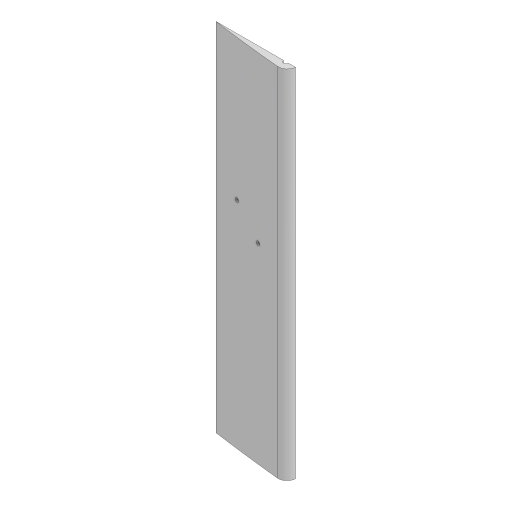
# Autodesk Inventor part: 5P.00.03.01-IB-VTP-Rudder-Right
Saved by Autodesk Inventor 2024.3 (Build 283343000, 343)
## iProperties
Created: 2024-11-01
Part Number: 5P.00.03.01-IB-VTP-Rudder-Right
Material: Generic
Document SubType Name: Modeling
Designer: inigo
Density: 1 g/cm^3
Appearance: Default
Author: inigo
Autodesk Inventor part; units mm, degrees
sketch "Sketch9" plane through (0, 0, 0) normal (0, 1, 0) x (-1, 0, 0)
  spline S0 degree 4 poles (158.6, 0) (158.582, 0.0027) (158.4943, 0.0152) (158.3472, 0.0367) (158.0986, 0.0728) (157.8372, 0.1103) (157.5162, 0.1567) (157.1379, 0.2109) (156.7024, 0.273) (156.2099, 0.3431) (155.661, 0.4204) (155.0564, 0.5055) (154.3967, 0.5974) (153.6823, 0.6963) (152.9144, 0.8018) (152.0931, 0.9136) (151.2197, 1.0314) (150.2949, 1.1553) (149.3195, 1.2842) (148.2947, 1.4185) (147.2214, 1.5576) (146.1008, 1.7014) (144.9336, 1.8489) (143.7214, 2.0008) (142.465, 2.156) (141.166, 2.3142) (139.8256, 2.4755) (138.445, 2.6392) (137.0256, 2.8051) (135.5689, 2.9729) (134.0761, 3.1422) (132.5489, 3.3123) (130.9887, 3.4837) (129.3972, 3.6552) (127.7758, 3.827) (126.126, 3.9983) (124.4499, 4.1692) (122.7486, 4.3392) (121.024, 4.5076) (119.2779, 4.6746) (117.5118, 4.8392) (115.7279, 5.0016) (113.9273, 5.1612) (112.1123, 5.3173) (110.2844, 5.47) (108.4455, 5.6184) (106.5976, 5.7628) (104.7421, 5.9018) (102.8813, 6.0361) (101.0167, 6.1642) (99.1503, 6.2867) (97.2839, 6.4023) (95.4193, 6.511) (93.5585, 6.6124) (91.703, 6.7063) (89.8551, 6.7915) (88.0161, 6.8687) (86.1882, 6.9365) (84.3732, 6.9953) (82.5726, 7.0442) (80.7886, 7.0832) (79.0224, 7.1119) (77.2764, 7.1298) (75.5517, 7.1371) (73.8503, 7.133) (72.1741, 7.1177) (70.5243, 7.091) (68.9027, 7.0524) (67.3112, 7.0021) (65.7508, 6.94) (64.2236, 6.8657) (62.7307, 6.7798) (61.2739, 6.6817) (59.8543, 6.5718) (58.4735, 6.4501) (57.133, 6.3171) (55.8338, 6.1722) (54.5772, 6.0162) (53.3648, 5.8493) (52.1973, 5.6715) (51.0764, 5.483) (50.0027, 5.2845) (48.9775, 5.0759) (48.0018, 4.858) (47.0765, 4.6308) (46.2025, 4.3948) (45.3805, 4.1502) (44.6117, 3.8978) (43.8963, 3.6374) (43.2353, 3.3698) (42.6292, 3.095) (42.0785, 2.8136) (41.5834, 2.526) (41.1451, 2.2317) (40.7628, 1.9317) (40.4377, 1.6254) (40.1698, 1.3127) (39.9596, 0.9936) (39.8087, 0.6678) (39.7177, 0.3364) (39.6875, 0) (39.7177, -0.3364) (39.8087, -0.6678) (39.9596, -0.9936) (40.1698, -1.3127) (40.4377, -1.6254) (40.7628, -1.9317) (41.1451, -2.2317) (41.5834, -2.526) (42.0785, -2.8136) (42.6292, -3.095) (43.2353, -3.3698) (43.8963, -3.6374) (44.6117, -3.8978) (45.3805, -4.1502) (46.2025, -4.3948) (47.0765, -4.6308) (48.0018, -4.858) (48.9775, -5.0759) (50.0027, -5.2845) (51.0764, -5.483) (52.1973, -5.6715) (53.3648, -5.8493) (54.5772, -6.0162) (55.8338, -6.1722) (57.133, -6.3171) (58.4735, -6.4501) (59.8543, -6.5718) (61.2739, -6.6817) (62.7307, -6.7798) (64.2236, -6.8657) (65.7508, -6.94) (67.3112, -7.0021) (68.9027, -7.0524) (70.5243, -7.091) (72.1741, -7.1177) (73.8503, -7.133) (75.5517, -7.1371) (77.2764, -7.1298) (79.0224, -7.1119) (80.7886, -7.0832) (82.5726, -7.0442) (84.3732, -6.9953) (86.1882, -6.9365) (88.0161, -6.8687) (89.8551, -6.7915) (91.703, -6.7063) (93.5585, -6.6124) (95.4193, -6.511) (97.2839, -6.4023) (99.1503, -6.2867) (101.0167, -6.1642) (102.8813, -6.0361) (104.7421, -5.9018) (106.5976, -5.7628) (108.4455, -5.6184) (110.2844, -5.47) (112.1123, -5.3173) (113.9273, -5.1612) (115.7279, -5.0016) (117.5118, -4.8392) (119.2779, -4.6746) (121.024, -4.5076) (122.7486, -4.3392) (124.4499, -4.1692) (126.126, -3.9983) (127.7758, -3.827) (129.3972, -3.6552) (130.9887, -3.4837) (132.5489, -3.3123) (134.0761, -3.1422) (135.5689, -2.9729) (137.0256, -2.8051) (138.445, -2.6392) (139.8256, -2.4755) (141.166, -2.3142) (142.465, -2.156) (143.7214, -2.0008) (144.9336, -1.8489) (146.1008, -1.7014) (147.2214, -1.5576) (148.2947, -1.4185) (149.3195, -1.2842) (150.2949, -1.1553) (151.2197, -1.0314) (152.0931, -0.9136) (152.9144, -0.8018) (153.6823, -0.6963) (154.3967, -0.5974) (155.0564, -0.5055) (155.661, -0.4204) (156.2099, -0.3431) (156.7024, -0.273) (157.1379, -0.2109) (157.5162, -0.1567) (157.8372, -0.1103) (158.0986, -0.0728) (158.3472, -0.0367) (158.4943, -0.0152) (158.582, -0.0027) (158.6, 0) knots 0 0 0 0 0 0.003305 0.005251 0.007517 0.010057 0.012844 0.015853 0.019069 0.022477 0.026064 0.029821 0.033738 0.037807 0.04202 0.046371 0.050853 0.05546 0.060186 0.065027 0.069976 0.07503 0.080184 0.085434 0.090774 0.096201 0.101711 0.1073 0.112964 0.118699 0.124501 0.130368 0.136295 0.142278 0.148315 0.154402 0.160535 0.166711 0.172927 0.179179 0.185465 0.19178 0.198121 0.204486 0.210871 0.217273 0.223689 0.230115 0.236548 0.242985 0.249423 0.255859 0.262289 0.268711 0.275121 0.281516 0.287892 0.294248 0.300579 0.306882 0.313155 0.319394 0.325595 0.331757 0.337875 0.343946 0.349967 0.355935 0.361846 0.367698 0.373486 0.379209 0.384861 0.390441 0.395943 0.401366 0.406705 0.411957 0.417118 0.422185 0.427153 0.432019 0.436778 0.441428 0.445964 0.450381 0.454676 0.458845 0.462884 0.466789 0.470556 0.474184 0.477671 0.481017 0.484224 0.487301 0.490258 0.493116 0.495899 0.498638 0.501362 0.504101 0.506884 0.509742 0.512699 0.515776 0.518983 0.522329 0.525816 0.529444 0.533211 0.537116 0.541155 0.545324 0.549619 0.554036 0.558572 0.563222 0.567981 0.572847 0.577815 0.582882 0.588043 0.593295 0.598634 0.604057 0.609559 0.615139 0.620791 0.626514 0.632302 0.638154 0.644065 0.650033 0.656054 0.662125 0.668243 0.674405 0.680606 0.686845 0.693118 0.699421 0.705752 0.712108 0.718484 0.724879 0.731289 0.737711 0.744141 0.750577 0.757015 0.763452 0.769885 0.776311 0.782727 0.789129 0.795514 0.801879 0.80822 0.814535 0.820821 0.827073 0.833289 0.839465 0.845598 0.851685 0.857722 0.863705 0.869632 0.875499 0.881301 0.887036 0.8927 0.898289 0.903799 0.909226 0.914566 0.919816 0.92497 0.930024 0.934973 0.939814 0.94454 0.949147 0.953629 0.95798 0.962193 0.966262 0.970179 0.973936 0.977523 0.980931 0.984147 0.987156 0.989943 0.992483 0.994749 0.996695 1 1 1 1 1
  point P0 (158.4826, 0.017)
  point P1 (158.3362, 0.0383)
  point P2 (158.1312, 0.068)
  point P3 (157.8681, 0.1059)
  point P4 (157.547, 0.1522)
  point P5 (157.1682, 0.2065)
  point P6 (156.7323, 0.2687)
  point P7 (156.2395, 0.3387)
  point P8 (155.6903, 0.4163)
  point P9 (155.0853, 0.5013)
  point P10 (154.4252, 0.5933)
  point P11 (153.7105, 0.6922)
  point P12 (152.942, 0.7978)
  point P13 (152.1203, 0.9097)
  point P14 (151.2464, 1.0277)
  point P15 (150.3211, 1.1514)
  point P16 (149.3453, 1.2806)
  point P17 (148.3199, 1.4149)
  point P18 (147.246, 1.5541)
  point P19 (146.1248, 1.6979)
  point P20 (144.9571, 1.8457)
  point P21 (143.7442, 1.9975)
  point P22 (142.4871, 2.1528)
  point P23 (141.1875, 2.3112)
  point P24 (139.8464, 2.4725)
  point P25 (138.465, 2.6364)
  point P26 (137.0449, 2.8024)
  point P27 (135.5874, 2.9702)
  point P28 (134.0939, 3.1396)
  point P29 (132.5659, 3.3099)
  point P30 (131.0049, 3.4813)
  point P31 (129.4125, 3.653)
  point P32 (127.7903, 3.8248)
  point P33 (126.1397, 3.9962)
  point P34 (124.4626, 4.1672)
  point P35 (122.7604, 4.3372)
  point P36 (121.035, 4.5058)
  point P37 (119.288, 4.6728)
  point P38 (117.521, 4.8376)
  point P39 (115.7361, 5)
  point P40 (113.9346, 5.1595)
  point P41 (112.1187, 5.3158)
  point P42 (110.2899, 5.4684)
  point P43 (108.45, 5.6171)
  point P44 (106.6011, 5.7613)
  point P45 (104.7447, 5.9005)
  point P46 (102.8829, 6.0347)
  point P47 (101.0173, 6.1629)
  point P48 (99.15, 6.2853)
  point P49 (97.2827, 6.401)
  point P50 (95.4171, 6.5097)
  point P51 (93.5553, 6.6111)
  point P52 (91.6989, 6.7048)
  point P53 (89.85, 6.7901)
  point P54 (88.0101, 6.8671)
  point P55 (86.1813, 6.935)
  point P56 (84.3654, 6.9936)
  point P57 (82.5639, 7.0424)
  point P58 (80.779, 7.0813)
  point P59 (79.012, 7.1099)
  point P60 (77.265, 7.1277)
  point P61 (75.5396, 7.1347)
  point P62 (73.8374, 7.1306)
  point P63 (72.1603, 7.1151)
  point P64 (70.5097, 7.0881)
  point P65 (68.8875, 7.0493)
  point P66 (67.2951, 6.9988)
  point P67 (65.7341, 6.9364)
  point P68 (64.2061, 6.862)
  point P69 (62.7126, 6.7756)
  point P70 (61.2551, 6.6773)
  point P71 (59.835, 6.5671)
  point P72 (58.4536, 6.4451)
  point P73 (57.1125, 6.3116)
  point P74 (55.8129, 6.1664)
  point P75 (54.5558, 6.0099)
  point P76 (53.3429, 5.8425)
  point P77 (52.1752, 5.6642)
  point P78 (51.054, 5.4752)
  point P79 (49.9801, 5.2761)
  point P80 (48.9547, 5.0669)
  point P81 (47.9789, 4.8483)
  point P82 (47.0536, 4.6203)
  point P83 (46.1797, 4.3835)
  point P84 (45.358, 4.1381)
  point P85 (44.5895, 3.8846)
  point P86 (43.8748, 3.6232)
  point P87 (43.2147, 3.3545)
  point P88 (42.6097, 3.0787)
  point P89 (42.0605, 2.7962)
  point P90 (41.5677, 2.5074)
  point P91 (41.1318, 2.2124)
  point P92 (40.753, 1.9117)
  point P93 (40.4319, 1.6055)
  point P94 (40.1688, 1.2941)
  point P95 (39.9638, 0.9777)
  point P96 (39.8174, 0.6564)
  point P97 (39.7294, 0.3304)
  point P98 (39.7, 0)
  point P99 (39.7294, -0.3304)
  point P100 (39.8174, -0.6564)
  point P101 (39.9638, -0.9777)
  point P102 (40.1688, -1.2941)
  point P103 (40.4319, -1.6055)
  point P104 (40.753, -1.9117)
  point P105 (41.1318, -2.2124)
  point P106 (41.5677, -2.5074)
  point P107 (42.0605, -2.7962)
  point P108 (42.6097, -3.0787)
  point P109 (43.2147, -3.3545)
  point P110 (43.8748, -3.6232)
  point P111 (44.5895, -3.8846)
  point P112 (45.358, -4.1381)
  point P113 (46.1797, -4.3835)
  point P114 (47.0536, -4.6203)
  point P115 (47.9789, -4.8483)
  point P116 (48.9547, -5.0669)
  point P117 (49.9801, -5.2761)
  point P118 (51.054, -5.4752)
  point P119 (52.1752, -5.6642)
  point P120 (53.3429, -5.8425)
  point P121 (54.5558, -6.0099)
  point P122 (55.8129, -6.1664)
  point P123 (57.1125, -6.3116)
  point P124 (58.4536, -6.4451)
  point P125 (59.835, -6.5671)
  point P126 (61.2551, -6.6773)
  point P127 (62.7126, -6.7756)
  point P128 (64.2061, -6.862)
  point P129 (65.7341, -6.9364)
  point P130 (67.2951, -6.9988)
  point P131 (68.8875, -7.0493)
  point P132 (70.5097, -7.0881)
  point P133 (72.1603, -7.1151)
  point P134 (73.8374, -7.1306)
  point P135 (75.5396, -7.1347)
  point P136 (77.265, -7.1277)
  point P137 (79.012, -7.1099)
  point P138 (80.779, -7.0813)
  point P139 (82.5639, -7.0424)
  point P140 (84.3654, -6.9936)
  point P141 (86.1813, -6.935)
  point P142 (88.0101, -6.8671)
  point P143 (89.85, -6.7901)
  point P144 (91.6989, -6.7048)
  point P145 (93.5553, -6.6111)
  point P146 (95.4171, -6.5097)
  point P147 (97.2827, -6.401)
  point P148 (99.15, -6.2853)
  point P149 (101.0173, -6.1629)
  point P150 (102.8829, -6.0347)
  point P151 (104.7447, -5.9005)
  point P152 (106.6011, -5.7613)
  point P153 (108.45, -5.6171)
  point P154 (110.2899, -5.4684)
  point P155 (112.1187, -5.3158)
  point P156 (113.9346, -5.1595)
  point P157 (115.7361, -5)
  point P158 (117.521, -4.8376)
  point P159 (119.288, -4.6728)
  point P160 (121.035, -4.5058)
  point P161 (122.7604, -4.3372)
  point P162 (124.4626, -4.1672)
  point P163 (126.1397, -3.9962)
  point P164 (127.7903, -3.8248)
  point P165 (129.4125, -3.653)
  point P166 (131.0049, -3.4813)
  point P167 (132.5659, -3.3099)
  point P168 (134.0939, -3.1396)
  point P169 (135.5874, -2.9702)
  point P170 (137.0449, -2.8024)
  point P171 (138.465, -2.6364)
  point P172 (139.8464, -2.4725)
  point P173 (141.1875, -2.3112)
  point P174 (142.4871, -2.1528)
  point P175 (143.7442, -1.9975)
  point P176 (144.9571, -1.8457)
  point P177 (146.1248, -1.6979)
  point P178 (147.246, -1.5541)
  point P179 (148.3199, -1.4149)
  point P180 (149.3453, -1.2806)
  point P181 (150.3211, -1.1514)
  point P182 (151.2464, -1.0277)
  point P183 (152.1203, -0.9097)
  point P184 (152.942, -0.7978)
  point P185 (153.7105, -0.6922)
  point P186 (154.4252, -0.5933)
  point P187 (155.0853, -0.5013)
  point P188 (155.6903, -0.4163)
  point P189 (156.2395, -0.3387)
  point P190 (156.7323, -0.2687)
  point P191 (157.1682, -0.2065)
  point P192 (157.547, -0.1522)
  point P193 (157.8681, -0.1059)
  point P194 (158.1312, -0.068)
  point P195 (158.3362, -0.0383)
  point P196 (158.4826, -0.017)
  point P197 (158.5706, -0.0043)
  constraints: 201 other
ref_plane "Work Plane4" through (0, -250, 0) normal (0, 1, 0) x (-1, 0, 0)
sketch "Sketch10" plane through (0, -250, 0) normal (0, 1, 0) x (-1, 0, 0)
  spline S0 degree 4 poles (158.6, 0) (158.576, 0.0036) (158.459, 0.0203) (158.2628, 0.049) (157.9312, 0.0971) (157.5825, 0.1472) (157.1543, 0.209) (156.6498, 0.2814) (156.0688, 0.3641) (155.4118, 0.4577) (154.6797, 0.5608) (153.8733, 0.6743) (152.9932, 0.7968) (152.0404, 0.9287) (151.016, 1.0695) (149.9204, 1.2187) (148.7554, 1.3758) (147.5218, 1.541) (146.2209, 1.713) (144.8539, 1.8922) (143.4221, 2.0777) (141.9274, 2.2695) (140.3704, 2.4662) (138.7535, 2.6689) (137.0777, 2.8758) (135.3449, 3.0868) (133.557, 3.3021) (131.7153, 3.5205) (129.822, 3.7417) (127.8789, 3.9656) (125.8877, 4.1913) (123.8507, 4.4183) (121.7694, 4.6469) (119.6466, 4.8756) (117.4838, 5.1049) (115.2832, 5.3332) (113.0473, 5.5613) (110.778, 5.788) (108.4775, 6.0127) (106.1485, 6.2354) (103.7927, 6.455) (101.4131, 6.6716) (99.0113, 6.8844) (96.5903, 7.0927) (94.1522, 7.2964) (91.6992, 7.4944) (89.2343, 7.687) (86.7593, 7.8723) (84.2771, 8.0516) (81.7899, 8.2223) (79.3004, 8.3858) (76.8109, 8.54) (74.3237, 8.685) (71.8415, 8.8203) (69.3665, 8.9455) (66.9015, 9.0592) (64.4486, 9.1621) (62.0104, 9.2526) (59.5893, 9.331) (57.1875, 9.3962) (54.8079, 9.4483) (52.452, 9.4866) (50.1229, 9.5104) (47.8224, 9.5201) (45.5529, 9.5147) (43.317, 9.4943) (41.1163, 9.4586) (38.9534, 9.4071) (36.8304, 9.34) (34.7491, 9.2572) (32.7119, 9.1581) (30.7205, 9.0435) (28.7773, 8.9126) (26.8838, 8.7661) (25.0419, 8.6037) (23.2537, 8.4263) (21.5207, 8.2331) (19.8446, 8.0249) (18.2273, 7.8024) (16.6701, 7.5651) (15.175, 7.3138) (13.7428, 7.049) (12.3753, 6.7708) (11.0737, 6.4801) (9.8395, 6.177) (8.6736, 5.8622) (7.5772, 5.536) (6.5516, 5.1992) (5.5974, 4.8518) (4.7157, 4.4949) (3.9072, 4.1284) (3.1726, 3.753) (2.5123, 3.3694) (1.9276, 2.9769) (1.4176, 2.5767) (0.984, 2.1681) (0.6267, 1.751) (0.3463, 1.3254) (0.1449, 0.8908) (0.0236, 0.4487) (-0.0167, 0) (0.0236, -0.4487) (0.1449, -0.8908) (0.3463, -1.3254) (0.6267, -1.751) (0.984, -2.1681) (1.4176, -2.5767) (1.9276, -2.9769) (2.5123, -3.3694) (3.1726, -3.753) (3.9072, -4.1284) (4.7157, -4.4949) (5.5974, -4.8518) (6.5516, -5.1992) (7.5772, -5.536) (8.6736, -5.8622) (9.8395, -6.177) (11.0737, -6.4801) (12.3753, -6.7708) (13.7428, -7.049) (15.175, -7.3138) (16.6701, -7.5651) (18.2273, -7.8024) (19.8446, -8.0249) (21.5207, -8.2331) (23.2537, -8.4263) (25.0419, -8.6037) (26.8838, -8.7661) (28.7773, -8.9126) (30.7205, -9.0435) (32.7119, -9.1581) (34.7491, -9.2572) (36.8304, -9.34) (38.9534, -9.4071) (41.1163, -9.4586) (43.317, -9.4943) (45.5529, -9.5147) (47.8224, -9.5201) (50.1229, -9.5104) (52.452, -9.4866) (54.8079, -9.4483) (57.1875, -9.3962) (59.5893, -9.331) (62.0104, -9.2526) (64.4486, -9.1621) (66.9015, -9.0592) (69.3665, -8.9455) (71.8415, -8.8203) (74.3237, -8.685) (76.8109, -8.54) (79.3004, -8.3858) (81.7899, -8.2223) (84.2771, -8.0516) (86.7593, -7.8723) (89.2343, -7.687) (91.6992, -7.4944) (94.1522, -7.2964) (96.5903, -7.0927) (99.0113, -6.8844) (101.4131, -6.6716) (103.7927, -6.455) (106.1485, -6.2354) (108.4775, -6.0127) (110.778, -5.788) (113.0473, -5.5613) (115.2832, -5.3332) (117.4838, -5.1049) (119.6466, -4.8756) (121.7694, -4.6469) (123.8507, -4.4183) (125.8877, -4.1913) (127.8789, -3.9656) (129.822, -3.7417) (131.7153, -3.5205) (133.557, -3.3021) (135.3449, -3.0868) (137.0777, -2.8758) (138.7535, -2.6689) (140.3704, -2.4662) (141.9274, -2.2695) (143.4221, -2.0777) (144.8539, -1.8922) (146.2209, -1.713) (147.5218, -1.541) (148.7554, -1.3758) (149.9204, -1.2187) (151.016, -1.0695) (152.0404, -0.9287) (152.9932, -0.7968) (153.8733, -0.6743) (154.6797, -0.5608) (155.4118, -0.4577) (156.0688, -0.3641) (156.6498, -0.2814) (157.1543, -0.209) (157.5825, -0.1472) (157.9312, -0.0971) (158.2628, -0.049) (158.459, -0.0203) (158.576, -0.0036) (158.6, 0) knots 0 0 0 0 0 0.003305 0.005251 0.007517 0.010057 0.012844 0.015853 0.019069 0.022477 0.026064 0.029821 0.033738 0.037807 0.04202 0.046371 0.050853 0.05546 0.060186 0.065027 0.069976 0.07503 0.080184 0.085434 0.090774 0.096201 0.101711 0.1073 0.112964 0.118699 0.124501 0.130368 0.136295 0.142278 0.148315 0.154402 0.160535 0.166711 0.172927 0.179179 0.185465 0.19178 0.198121 0.204486 0.210871 0.217273 0.223689 0.230115 0.236548 0.242985 0.249423 0.255859 0.262289 0.268711 0.275121 0.281516 0.287892 0.294248 0.300579 0.306882 0.313155 0.319394 0.325595 0.331757 0.337875 0.343946 0.349967 0.355935 0.361846 0.367698 0.373486 0.379209 0.384861 0.390441 0.395943 0.401366 0.406705 0.411957 0.417118 0.422185 0.427153 0.432019 0.436778 0.441428 0.445964 0.450381 0.454676 0.458845 0.462884 0.466789 0.470556 0.474184 0.477671 0.481017 0.484224 0.487301 0.490258 0.493116 0.495899 0.498638 0.501362 0.504101 0.506884 0.509742 0.512699 0.515776 0.518983 0.522329 0.525816 0.529444 0.533211 0.537116 0.541155 0.545324 0.549619 0.554036 0.558572 0.563222 0.567981 0.572847 0.577815 0.582882 0.588043 0.593295 0.598634 0.604057 0.609559 0.615139 0.620791 0.626514 0.632302 0.638154 0.644065 0.650033 0.656054 0.662125 0.668243 0.674405 0.680606 0.686845 0.693118 0.699421 0.705752 0.712108 0.718484 0.724879 0.731289 0.737711 0.744141 0.750577 0.757015 0.763452 0.769885 0.776311 0.782727 0.789129 0.795514 0.801879 0.80822 0.814535 0.820821 0.827073 0.833289 0.839465 0.845598 0.851685 0.857722 0.863705 0.869632 0.875499 0.881301 0.887036 0.8927 0.898289 0.903799 0.909226 0.914566 0.919816 0.92497 0.930024 0.934973 0.939814 0.94454 0.949147 0.953629 0.95798 0.962193 0.966262 0.970179 0.973936 0.977523 0.980931 0.984147 0.987156 0.989943 0.992483 0.994749 0.996695 1 1 1 1 1
  point P0 (0, 0)
  point P1 (158.4435, 0.0227)
  point P2 (158.2481, 0.0511)
  point P3 (157.9746, 0.0907)
  point P4 (157.6237, 0.1413)
  point P5 (157.1954, 0.203)
  point P6 (156.6901, 0.2755)
  point P7 (156.1087, 0.3584)
  point P8 (155.4513, 0.4519)
  point P9 (154.7187, 0.5553)
  point P10 (153.9118, 0.6687)
  point P11 (153.0312, 0.7914)
  point P12 (152.0779, 0.9234)
  point P13 (151.0529, 1.0642)
  point P14 (149.9568, 1.2134)
  point P15 (148.7911, 1.3708)
  point P16 (147.5568, 1.5359)
  point P17 (146.2552, 1.7081)
  point P18 (144.8874, 1.8873)
  point P19 (143.455, 2.0731)
  point P20 (141.9594, 2.2648)
  point P21 (140.4018, 2.4619)
  point P22 (138.7839, 2.6645)
  point P23 (137.1072, 2.8716)
  point P24 (135.3735, 3.0829)
  point P25 (133.5847, 3.2981)
  point P26 (131.742, 3.5166)
  point P27 (129.8477, 3.738)
  point P28 (127.9036, 3.962)
  point P29 (125.9114, 4.1878)
  point P30 (123.8733, 4.4151)
  point P31 (121.791, 4.6436)
  point P32 (119.667, 4.8727)
  point P33 (117.5031, 5.1018)
  point P34 (115.3014, 5.3305)
  point P35 (113.0644, 5.5586)
  point P36 (110.7938, 5.7854)
  point P37 (108.4922, 6.0103)
  point P38 (106.1619, 6.233)
  point P39 (103.805, 6.4528)
  point P40 (101.4241, 6.6694)
  point P41 (99.0211, 6.8823)
  point P42 (96.5988, 7.0907)
  point P43 (94.1594, 7.2943)
  point P44 (91.7052, 7.4926)
  point P45 (89.239, 7.685)
  point P46 (86.7628, 7.8707)
  point P47 (84.2792, 8.0496)
  point P48 (81.7908, 8.2207)
  point P49 (79.3, 8.3839)
  point P50 (76.8092, 8.5382)
  point P51 (74.3208, 8.6832)
  point P52 (71.8372, 8.8185)
  point P53 (69.361, 8.9435)
  point P54 (66.8948, 9.0573)
  point P55 (64.4406, 9.1599)
  point P56 (62.0012, 9.2505)
  point P57 (59.5789, 9.3287)
  point P58 (57.1759, 9.3939)
  point P59 (54.795, 9.4457)
  point P60 (52.4381, 9.4838)
  point P61 (50.1078, 9.5076)
  point P62 (47.8062, 9.517)
  point P63 (45.5356, 9.5114)
  point P64 (43.2986, 9.4908)
  point P65 (41.0969, 9.4548)
  point P66 (38.933, 9.4031)
  point P67 (36.809, 9.3357)
  point P68 (34.7267, 9.2524)
  point P69 (32.6886, 9.1531)
  point P70 (30.6964, 9.038)
  point P71 (28.7523, 8.9068)
  point P72 (26.858, 8.7598)
  point P73 (25.0153, 8.5971)
  point P74 (23.2265, 8.419)
  point P75 (21.4928, 8.2253)
  point P76 (19.8161, 8.0166)
  point P77 (18.1982, 7.7933)
  point P78 (16.6406, 7.5554)
  point P79 (15.145, 7.3034)
  point P80 (13.7126, 7.0377)
  point P81 (12.3448, 6.7587)
  point P82 (11.0432, 6.4671)
  point P83 (9.8089, 6.163)
  point P84 (8.6432, 5.8471)
  point P85 (7.5471, 5.5198)
  point P86 (6.5221, 5.1816)
  point P87 (5.5688, 4.833)
  point P88 (4.6882, 4.4746)
  point P89 (3.8813, 4.1066)
  point P90 (3.1487, 3.7298)
  point P91 (2.4913, 3.3446)
  point P92 (1.9099, 2.9511)
  point P93 (1.4046, 2.55)
  point P94 (0.9763, 2.1416)
  point P95 (0.6254, 1.7262)
  point P96 (0.3519, 1.3042)
  point P97 (0.1565, 0.8756)
  point P98 (0.0392, 0.4407)
  point P99 (0, 0)
  point P100 (0.0392, -0.4407)
  point P101 (0.1565, -0.8756)
  point P102 (0.3519, -1.3042)
  point P103 (0.6254, -1.7262)
  point P104 (0.9763, -2.1416)
  point P105 (1.4046, -2.55)
  point P106 (1.9099, -2.9511)
  point P107 (2.4913, -3.3446)
  point P108 (3.1487, -3.7298)
  point P109 (3.8813, -4.1066)
  point P110 (4.6882, -4.4746)
  point P111 (5.5688, -4.833)
  point P112 (6.5221, -5.1816)
  point P113 (7.5471, -5.5198)
  point P114 (8.6432, -5.8471)
  point P115 (9.8089, -6.163)
  point P116 (11.0432, -6.4671)
  point P117 (12.3448, -6.7587)
  point P118 (13.7126, -7.0377)
  point P119 (15.145, -7.3034)
  point P120 (16.6406, -7.5554)
  point P121 (18.1982, -7.7933)
  point P122 (19.8161, -8.0166)
  point P123 (21.4928, -8.2253)
  point P124 (23.2265, -8.419)
  point P125 (25.0153, -8.5971)
  point P126 (26.858, -8.7598)
  point P127 (28.7523, -8.9068)
  point P128 (30.6964, -9.038)
  point P129 (32.6886, -9.1531)
  point P130 (34.7267, -9.2524)
  point P131 (36.809, -9.3357)
  point P132 (38.933, -9.4031)
  point P133 (41.0969, -9.4548)
  point P134 (43.2986, -9.4908)
  point P135 (45.5356, -9.5114)
  point P136 (47.8062, -9.517)
  point P137 (50.1078, -9.5076)
  point P138 (52.4381, -9.4838)
  point P139 (54.795, -9.4457)
  point P140 (57.1759, -9.3939)
  point P141 (59.5789, -9.3287)
  point P142 (62.0012, -9.2505)
  point P143 (64.4406, -9.1599)
  point P144 (66.8948, -9.0573)
  point P145 (69.361, -8.9435)
  point P146 (71.8372, -8.8185)
  point P147 (74.3208, -8.6832)
  point P148 (76.8092, -8.5382)
  point P149 (79.3, -8.3839)
  point P150 (81.7908, -8.2207)
  point P151 (84.2792, -8.0496)
  point P152 (86.7628, -7.8707)
  point P153 (89.239, -7.685)
  point P154 (91.7052, -7.4926)
  point P155 (94.1594, -7.2943)
  point P156 (96.5988, -7.0907)
  point P157 (99.0211, -6.8823)
  point P158 (101.4241, -6.6694)
  point P159 (103.805, -6.4528)
  point P160 (106.1619, -6.233)
  point P161 (108.4922, -6.0103)
  point P162 (110.7938, -5.7854)
  point P163 (113.0644, -5.5586)
  point P164 (115.3014, -5.3305)
  point P165 (117.5031, -5.1018)
  point P166 (119.667, -4.8727)
  point P167 (121.791, -4.6436)
  point P168 (123.8733, -4.4151)
  point P169 (125.9114, -4.1878)
  point P170 (127.9036, -3.962)
  point P171 (129.8477, -3.738)
  point P172 (131.742, -3.5166)
  point P173 (133.5847, -3.2981)
  point P174 (135.3735, -3.0829)
  point P175 (137.1072, -2.8716)
  point P176 (138.7839, -2.6645)
  point P177 (140.4018, -2.4619)
  point P178 (141.9594, -2.2648)
  point P179 (143.455, -2.0731)
  point P180 (144.8874, -1.8873)
  point P181 (146.2552, -1.7081)
  point P182 (147.5568, -1.5359)
  point P183 (148.7911, -1.3708)
  point P184 (149.9568, -1.2134)
  point P185 (151.0529, -1.0642)
  point P186 (152.0779, -0.9234)
  point P187 (153.0312, -0.7914)
  point P188 (153.9118, -0.6687)
  point P189 (154.7187, -0.5553)
  point P190 (155.4513, -0.4519)
  point P191 (156.1087, -0.3584)
  point P192 (156.6901, -0.2755)
  point P193 (157.1954, -0.203)
  point P194 (157.6237, -0.1413)
  point P195 (157.9746, -0.0907)
  point P196 (158.2481, -0.0511)
  point P197 (158.4435, -0.0227)
  point P198 (158.5608, -0.0057)
  constraints: 201 other
loft "Loft3" add profiles "Sketch10", "Sketch9"
ref_plane "Work Plane5" through (0, 10, 0) normal (0, 1, 0) x (-1, 0, 0)
ref_plane "Work Plane8" through (-109.1, 0, 0) normal (1, 0, 0) x (0, 1, 0)
ref_plane "Work Plane7" through (-158.6, 0, 0) normal (1, 0, 0) x (0, 1, 0)
split "Split4" plane through (-109.1, 0, 0) removes the side toward (1, 0, 0)
ref_plane "Work Plane9" through (-109.1, -22, 5.5651) normal (0, 1, 0) x (1, 0, 0)
split "Split5" plane through (-109.1, -22, 5.5651) removes the side toward (0, 1, 0)
fillet "Fillet1" radius 5.5 2 edges at (-109.1, -136, 5.8042) (-109.1, -136, -5.8042)
sketch "Sketch23" plane through (-109.1, -22, 5.5651) normal (0, 1, 0) x (1, 0, 0)
  circle A0 centre (-6, 5.5651) radius 1.5
  point P0 (109.1, 5.5651)
  point P1 (-49.5, 5.5651)
  dimension "d117" = 3
  dimension "d118" = 43.5
  constraints: 1 centre point
  measures "d117" diameter of A0
  measures "d118" distance of point (-49.5, 5.565) A0.centre
extrude "Extrusion14" cut sketch "Sketch23" against normal blind 230
split "Split6" plane through (0, 0, 0) removes the side toward (0, 0, -1)
ref_plane "Work Plane10" through (-158.6, -25, 0) normal (0, 1, 0) x (1, 0, 0)
split "Split7" plane through (-158.6, -25, 0) removes the side toward (0, 1, 0)
ref_plane "Work Plane11" through (-158.6, -247, 0) normal (0, -1, 0) x (1, 0, 0)
split "Split8" plane through (-158.6, -247, 0) removes the side toward (0, -1, 0)
sketch "Sketch24" plane through (-116.6, -25, 0) normal (0, 0, -1) x (-1, 0, 0)
  line L0 (0, -222) -> (42, -222) projected
  line L1 (42, -222) -> (42, 0) projected
  point P0 (-116.6, 25)
  point P1 (27, -87.8)
  point P2 (12, -102.8)
  dimension "d123" = 134.2
  dimension "d124" = 15
  dimension "d125" = 15
  dimension "d126" = 15
  measures "d123" distance from line of L0 point (27, -87.8)
  measures "d124" distance from line of L1 point (27, -87.8)
  measures "d125" horizontal distance of point (12, -102.8) point (27, -87.8)
  measures "d126" horizontal distance of point (12, -102.8) point (27, -87.8)
hole "Hole1" at (-143.6, -112.8, 0) at (-128.6, -127.8, 0) direction (0, 0, 1) diameter 2.4 depth 17.1 clearance for "Flat Head Machine Screw" size "M2" standard "Ansi Metric M Profile"
equation "\"rudHingeSeatLength\" = 18.985"
equation "\"rudLength\" = vtpLength - 2 * rudHingeSeatLength"
equation "\"rudWidth\" = 49.5"
equation "\"rootChord\" = 185"
equation "\"rudTurnRoom\" = 2.5"
equation "\"rudSpace\" = rudWidth + rudTurnRoom"
equation "\"d54\" = d57 - 2 * d56"
equation "\"d55\" = d58 + d59"
equation "\"d56\" = 18.985"
equation "\"d58\" = 49.5"
equation "\"d59\" = 2.5"
equation "\"sparDiam\" = 7"
equation "\"vtpLength\" = 250"
equation "\"d57\" = 250"
